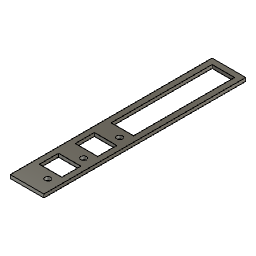
TV Cabinet Rack Posts (Autodesk Fusion 360 design; units mm, degrees)
Autodesk Fusion 360 part; units mm, degrees
sketch "Sketch1" plane through (0, 0, 0) normal (0, 0, 1) x (1, 0, 0) in component "Top-RIght-Front2"
  line L0 (0, 0) -> (-20, 0)
  line L1 (-20, 0) -> (-20, -180)
  line L2 (-20, -180) -> (0, -180)
  line L3 (0, -180) -> (0, 0)
  dimension "d41" = 20
  dimension "d42" = 180
  constraint horizontal L0
  constraint vertical L1
  constraint horizontal L2
  constraint vertical L3
  constraint coincident L0.start L3.end
  measures "d41" distance of L0.start L0.end
  measures "d42" distance of L0.start L2.end
sketch "Sketch2" plane through (0, 0, 0) normal (0, 0, 1) x (1, 0, 0) in component "Top-RIght-Front2"
  line L0 (0, 0) -> (10, 0)
  line L1 (10, 0) -> (10, -180)
  line L2 (10, -180) -> (0, -180)
  line L3 (0, -180) -> (0, 0)
  dimension "d43" = 10
  dimension "d44" = 180
  constraint horizontal L0
  constraint vertical L1
  constraint horizontal L2
  constraint vertical L3
  constraint coincident L0.start L3.end
  measures "d43" distance of L0.start L0.end
  measures "d44" distance of L0.start L2.end
extrude "Extrude1" add sketch "Sketch1" sketch "Sketch2" along normal blind 3 of sketch 2 in component "Top-RIght-Front2"
sketch "Sketch3" plane through (0, 0, 3) normal (0, 0, 1) x (-1, 0, 0) in component "Top-RIght-Front2"
  line L0 (-10, 0) -> (20, 0)
  line L1 (20, 0) -> (20, 180)
  line L2 (20, 180) -> (-10, 180)
  line L3 (-10, 180) -> (-10, 0)
  line L4 (0, 0) -> (0, 270) construction
  circle A0 centre (0, 102.5) radius 2.5
  dimension "d47" = 270
  dimension "d48" = 5
  dimension "d49" = 102.5
  constraint coincident L4.start origin
  constraint perpendicular L2 L4
  constraint coincident L4 A0.centre
  measures "d47" distance of L4.start L4.end
  measures "d48" diameter of A0
  measures "d49" distance of L4.start A0.centre
extrude "Extrude2" cut sketch "Sketch3" against normal up to surface (3 mm away) contours A0 in component "Top-RIght-Front2"
sketch "Sketch5" plane through (0, 0, 3) normal (0, 0, 1) x (-1, 0, 0) in component "Top-RIght-Front2"
  circle A0 centre (0, 102.5) radius 2.5
  line L0 (-10, 0) -> (20, 0)
  line L1 (20, 0) -> (20, 180)
  line L2 (20, 180) -> (-10, 180)
  line L3 (-10, 180) -> (-10, 0)
  line L4 (0, 0) -> (0, 227.7762) construction
  circle A1 centre (0, 134.5) radius 2.5
  circle A2 centre (0, 166.5) radius 2.5
  dimension "d52" = 5
  dimension "d53" = 32
  dimension "d54" = 5
  dimension "d55" = 32
  constraint coincident L4.start origin
  constraint perpendicular L0 L4
  constraint coincident L4 A1.centre
  constraint coincident L4 A2.centre
  measures "d52" diameter of A1
  measures "d53" distance of A0.centre A1.centre
  measures "d54" diameter of A2
  measures "d55" distance of A1.centre A2.centre
extrude "Extrude3" cut sketch "Sketch5" against normal up to surface (3 mm away) contours A1 | A2 in component "Top-RIght-Front2"
sketch "Sketch9" plane through (0, 0, 3) normal (0, 0, 1) x (-1, 0, 0) in component "Top-RIght-Front2"
  circle A0 centre (0, 134.5) radius 2.5
  circle A1 centre (0, 166.5) radius 2.5
  circle A2 centre (0, 102.5) radius 2.5
  line L0 (-10, 0) -> (20, 0)
  line L1 (20, 0) -> (20, 180)
  line L2 (20, 180) -> (-10, 180)
  line L3 (-10, 180) -> (-10, 0)
  line L4 (15, 5) -> (-5, 5)
  line L5 (-5, 5) -> (-5, 95)
  line L6 (-5, 95) -> (15, 95)
  line L7 (15, 95) -> (15, 5)
  line L8 (0, 0) -> (20, 0)
  line L9 (20, 0) -> (20, 180)
  line L10 (15, 110) -> (-5, 110)
  line L11 (-5, 110) -> (-5, 127)
  line L12 (-5, 127) -> (15, 127)
  line L13 (15, 127) -> (15, 110)
  line L14 (15, 142) -> (-5, 142)
  line L15 (-5, 142) -> (-5, 159)
  line L16 (-5, 159) -> (15, 159)
  line L17 (15, 159) -> (15, 142)
  dimension "d68" = 20
  dimension "d69" = 90
  dimension "d70" = 5
  dimension "d71" = 5
  dimension "d72" = 20
  dimension "d73" = 17
  dimension "d74" = 5
  dimension "d75" = 7.5
  dimension "d76" = 20
  dimension "d77" = 17
  dimension "d78" = 5
  dimension "d79" = 7.5
  constraint horizontal L4
  constraint vertical L5
  constraint horizontal L6
  constraint vertical L7
  constraint horizontal L10
  constraint vertical L11
  constraint horizontal L12
  constraint vertical L13
  constraint horizontal L14
  constraint vertical L15
  constraint horizontal L16
  constraint vertical L17
  measures "d68" distance of L4.start L4.end
  measures "d69" distance of L4.start L6.end
  measures "d70" distance of L4 L8
  measures "d71" distance of L7 L9
  measures "d72" distance of L10.start L10.end
  measures "d73" distance of L10.start L12.end
  measures "d74" distance of L3 L11
  measures "d75" distance of A2.centre L10
  measures "d76" distance of L14.start L14.end
  measures "d77" distance of L14.start L16.end
  measures "d78" distance of L3 L15
  measures "d79" distance of A0.centre L14
extrude "Extrude5" cut sketch "Sketch9" against normal up to surface (3 mm away) contours L4 L5 L6 L7 | L10 L11 L12 L13 | L14 L15 L16 L17 in component "Top-RIght-Front2"
component "Top-RIght-Front2" placed x (1, 0, 0) y (0, 1, 0) z (0, 0, 1) at (0, 0, 0)
